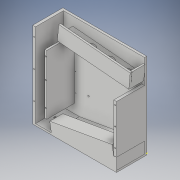
# Autodesk Inventor part: base part
Saved by Autodesk Inventor 2019 (Build 230136000, 136)
## iProperties
Created: 2020-02-20
Part Number: base part
Material: Generic
Document SubType Name: Modeling
Designer: LENOVO
Density: 1 g/cm^3
Appearance: Default
Author: LENOVO
Autodesk Inventor part; units mm, degrees
ref_plane "YZ Plane" through (0, 0, 0) normal (1, 0, 0) x (0, 1, 0)
ref_plane "XZ Plane" through (0, 0, 0) normal (0, 1, 0) x (-1, 0, 0)
ref_plane "XY Plane" through (0, 0, 0) normal (0, 0, 1) x (1, 0, 0)
sketch "Sketch1" plane through (0, 0, 0) normal (0, 0, 1) x (1, 0, 0)
  line L0 (0, 0) -> (450, 0)
  line L1 (450, 0) -> (450, 450)
  line L2 (450, 450) -> (0, 450)
  line L3 (0, 450) -> (0, 0)
  dimension "d0" = 450
  dimension "d1" = 450
  constraints: 8 end point, 2 parallel, 1 horizontal, 1 perpendicular
  measures "d0" distance of L2.end L1.end
  measures "d1" distance of L1.end L0.end
extrude "Extrusion1" add sketch "Sketch1" along normal blind 12
sketch "Sketch2" plane through (0, 0, 12) normal (0, 0, 1) x (1, 0, 0)
  line L0 (100, 400) -> (448.6681, 369.4955)
  line L1 (100, 400) -> (450, 400) construction
  line L2 (448.6681, 369.4955) -> (446.0535, 339.6096)
  line L3 (446.0535, 339.6096) -> (97.3853, 370.1142)
  line L4 (97.3853, 370.1142) -> (100, 400)
  point P0 (0, 0)
  dimension "d4" = 350
  dimension "d5" = 5
  dimension "d6" = 30
  dimension "d7" = 350
  constraints: 10 end point, 2 perpendicular, 1 equal length, 1 horizontal
  measures "d4" distance of L0.start L0.end
  measures "d5" angle of L0 L1
  measures "d6" distance of L0.end L2.end
  measures "d7" distance of L2.end L3.end
extrude "Extrusion2" add sketch "Sketch2" along normal blind 80
sketch "Sketch3" plane through (100, 400, 92) normal (0.0871557, 0.9961947, 0) x (0.9961947, -0.0871557, 0)
  circle A0 centre (100, 40) radius 25
  circle A1 centre (300, 40) radius 25
  circle A2 centre (200, 40) radius 25
  point P0 (-64.7572, 92)
  dimension "d10" = 50
  dimension "d11" = 50
  dimension "d12" = 50
  constraints: 3 centre point
  measures "d10" diameter of A0
  measures "d11" diameter of A1
  measures "d12" diameter of A2
extrude "Extrusion3" cut sketch "Sketch3" against normal blind 80
sketch "Sketch4" plane through (100, 400, 92) normal (0.0871557, 0.9961947, 0) x (0.9961947, -0.0871557, 0)
  line L0 (350, 0) -> (0, 0) projected
  line L1 (0, 0) -> (350, 0)
  line L2 (350, 0) -> (350, 10)
  line L3 (350, 10) -> (0, 10)
  line L4 (0, 10) -> (0, 0)
  point P0 (-64.7572, 92)
  dimension "d15" = 350
  dimension "d16" = 10
  constraints: 8 end point, 2 parallel, 1 horizontal, 1 perpendicular
  measures "d15" distance of L3.end L2.end
  measures "d16" distance of L2.end L1.end
extrude "Extrusion4" add sketch "Sketch4" along normal blind 50
sketch "Sketch5" plane through (0, 0, 0) normal (0, 0, -1) x (-1, 0, 0)
  point P0 (0, 0)
sketch "Sketch6" plane through (0, 0, 12) normal (0, 0, 1) x (1, 0, 0)
  circle A0 centre (135, 350) radius 6.5
  circle A1 centre (240, 345) radius 6.5
  circle A2 centre (340, 340) radius 6.5
  point P0 (0, 0)
  dimension "d19" = 13
  dimension "d20" = 13
  dimension "d21" = 13
  constraints: 3 centre point
  measures "d19" diameter of A0
  measures "d20" diameter of A1
  measures "d21" diameter of A2
extrude "Extrusion5" cut sketch "Sketch6" against normal blind 50
sketch "Sketch7" plane through (448.6681, 369.4955, 82) normal (0.0871557, 0.9961947, 0) x (0.9961947, -0.0871557, 0)
  line L0 (0, 70) -> (0, -10) projected
  line L1 (0, 0.4476) -> (-8.4239, 0.4476)
  line L2 (-8.4239, 0.4476) -> (-8.4239, 70)
  line L3 (-8.4239, 70) -> (0, 70)
  line L4 (0, 70) -> (0, 0.4476)
  point P0 (-414.7572, 82)
  constraints: 8 end point, 2 parallel, 1 horizontal, 1 perpendicular, 1 point on line
extrude "Extrusion6" add sketch "Sketch7" along normal blind 50
sketch "Sketch8" plane through (0, 0, 12) normal (0, 0, 1) x (1, 0, 0)
  line L0 (0, 0) -> (450, 0)
  line L1 (450, 0) -> (450, -50)
  line L2 (450, -50) -> (0, -50)
  line L3 (0, -50) -> (0, 0)
  dimension "d26" = 450
  dimension "d27" = 50
  constraints: 8 end point, 2 parallel, 1 horizontal, 1 perpendicular
  measures "d26" distance of L1.end L2.end
  measures "d27" distance of L0.end L1.end
extrude "Extrusion7" add sketch "Sketch8" against normal blind 12
sketch "Sketch9" plane through (0, 0, 12) normal (0, 0, 1) x (1, 0, 0)
  line L0 (450, 450) -> (0, 450) projected
  line L1 (100, 450) -> (100, 0)
  line L2 (100, 0) -> (449.6068, 61.6451)
  line L3 (449.6068, 61.6451) -> (449.6068, 0)
  line L4 (449.6068, 0) -> (100, 0)
  point P0 (0, 0)
  dimension "d30" = 355
  dimension "d31" = 80
  dimension "d32" = 80
  constraints: 8 end point, 1 perpendicular, 1 point on line, 1 vertical
  measures "d30" distance of L1.end L2.end
  measures "d31" angle of L2 L1
  measures "d32" angle of L2 L3
extrude "Extrusion8" add sketch "Sketch9" along normal blind 85
sketch "Sketch10" plane through (0, 0, 12) normal (0, 0, 1) x (1, 0, 0)
  line L0 (450, -50) -> (0, -50) projected
  line L1 (0, 0) -> (450, 0)
  line L2 (450, 0) -> (450, -50)
  line L3 (450, -50) -> (0, -50)
  line L4 (0, -50) -> (0, 0)
  constraints: 8 end point, 2 parallel, 1 horizontal, 1 perpendicular
sketch "Sketch11" plane through (0, 0, 97) normal (0, 0, 1) x (1, 0, 0)
  line L0 (100, 0) -> (449.6068, 0) projected
  line L1 (449.6068, 61.6451) -> (100, 0) projected
  line L2 (100, 0) -> (449.6068, 61.6451)
  line L3 (449.6068, 61.6451) -> (449.6068, 0)
  line L4 (449.6068, 0) -> (100, 0)
  point P0 (0, 0)
  constraints: 6 end point, 1 collinear, 1 perpendicular, 1 vertical
extrude "Extrusion9" add sketch "Sketch11" along normal blind 65
extrude "Extrusion10" add sketch "Sketch10" along normal blind 150
sketch "Sketch12" plane through (0, 0, 12) normal (0, 0, 1) x (1, 0, 0)
  line L0 (0, 450) -> (0, -50) projected
  line L1 (0, 0) -> (100, 0) projected
  line L2 (0, 450) -> (15, 450)
  line L3 (15, 450) -> (15, 0)
  line L4 (15, 0) -> (0, 0)
  line L5 (0, 0) -> (0, 450)
  line L6 (450, 384.7187) -> (450, 0) projected
  line L7 (450, 320) -> (435, 320)
  line L8 (435, 320) -> (435, 61)
  line L9 (435, 61) -> (450, 61)
  line L10 (450, 61) -> (450, 320)
  dimension "d39" = 15
  dimension "d40" = 15
  dimension "d41" = 259
  constraints: 16 end point, 4 parallel, 2 horizontal, 2 perpendicular, 2 point on line
  measures "d39" distance of L3.end L4.end
  measures "d40" distance of L9.end L8.end
  measures "d41" distance of L8.end L7.end
extrude "Extrusion11" add sketch "Sketch12" along normal blind 150
sketch "Sketch13" plane through (449.6068, 0, 162) normal (1, 0, 0) x (0, 0, -1)
  line L0 (150, 0) -> (0, 0) projected
  line L1 (150, 61) -> (0, 61) projected
  line L2 (0, 0) -> (150, 0)
  line L3 (150, 0) -> (150, 61)
  line L4 (150, 61) -> (0, 61)
  line L5 (0, 61) -> (0, 0)
  point P0 (162, 0)
  constraints: 8 end point, 2 parallel, 1 horizontal, 1 perpendicular
extrude "Extrusion12" add sketch "Sketch13" along normal blind 0.4
sketch "Sketch14" plane through (0, 0, 12) normal (0, 0, 1) x (1, 0, 0)
  line L0 (75, 370) -> (65, 370)
  line L1 (65, 370) -> (65, 50)
  line L2 (65, 50) -> (75, 50)
  line L3 (75, 50) -> (75, 370)
  point P0 (0, 0)
  dimension "d46" = 10
  dimension "d47" = 320
  constraints: 8 end point, 2 parallel, 1 horizontal, 1 perpendicular
  measures "d46" distance of L2.end L1.end
  measures "d47" distance of L1.end L0.end
extrude "Extrusion13" add sketch "Sketch14" along normal blind 150
sketch "Sketch15" plane through (100, 0, 162) normal (0, 1, 0) x (1, 0, 0)
  circle A0 centre (-60, 81) radius 6.5
  point P0 (-100, 162)
  dimension "d50" = 13
  constraints: 1 centre point
  measures "d50" diameter of A0
extrude "Extrusion14" cut sketch "Sketch15" against normal blind 150
thread "Thread1" size "M14x2" class "6H" standard "ANSI Metric M Profile" full length
sketch "Sketch16" plane through (100, 0, 162) normal (-0.1736482, 0.9848078, 0) x (0.9848078, 0.1736482, 0)
  line L0 (0, 150) -> (0, 0) projected
  line L1 (0, 0) -> (340, 0)
  line L2 (340, 0) -> (340, 70)
  line L3 (340, 70) -> (0, 70)
  line L4 (0, 70) -> (0, 0)
  point P0 (-98.4808, 162)
  dimension "d55" = 340
  dimension "d56" = 70
  constraints: 8 end point, 2 parallel, 1 horizontal, 1 perpendicular
  measures "d55" distance of L3.end L2.end
  measures "d56" distance of L2.end L1.end
extrude "Extrusion15" add sketch "Sketch16" along normal blind 50
sketch "Sketch17" plane through (0, -50, 0) normal (0, -1, 0) x (1, 0, 0)
  line L0 (450, 0) -> (0, 0) projected
  line L1 (0, 0) -> (450, 0)
  line L2 (450, 0) -> (450, 162)
  line L3 (450, 162) -> (0, 162)
  line L4 (0, 162) -> (0, 0)
  dimension "d59" = 450
  constraints: 8 end point, 2 parallel, 1 horizontal, 1 perpendicular
  measures "d59" distance of L3.end L2.end
extrude "Extrusion16" cut sketch "Sketch17" against normal blind 20
sketch "Sketch18" plane through (0, -30, 0) normal (0, -1, 0) x (1, 0, 0)
  line L0 (0, 0) -> (450, 0)
  line L1 (450, 0) -> (450, 162)
  line L2 (450, 162) -> (0, 162)
  line L3 (0, 162) -> (0, 0)
  dimension "d62" = 450
  dimension "d63" = 162
  constraints: 8 end point, 2 parallel, 1 horizontal, 1 perpendicular
  measures "d62" distance of L2.end L1.end
  measures "d63" distance of L1.end L0.end
extrude "Extrusion17" cut sketch "Sketch18" against normal blind 10
sketch "Sketch19" plane through (0, -20, 0) normal (0, -1, 0) x (1, 0, 0)
  line L0 (450, 12) -> (450, 162) projected
  line L1 (0, 0) -> (450, 0)
  line L2 (450, 0) -> (450, 162)
  line L3 (450, 162) -> (0, 162)
  line L4 (0, 162) -> (0, 0)
  constraints: 8 end point, 2 parallel, 1 horizontal, 1 perpendicular
extrude "Extrusion18" cut sketch "Sketch19" against normal blind 10
sketch "Sketch20" plane through (0, 0, 162) normal (0, 0, 1) x (1, 0, 0)
  circle A0 centre (70, 340) radius 3
  circle A1 centre (70, 100) radius 3
  circle A2 centre (70, 230) radius 3
  point P0 (0, 0)
  dimension "d68" = 6
  dimension "d69" = 6
  dimension "d70" = 6
  constraints: 3 centre point
  measures "d68" diameter of A0
  measures "d69" diameter of A1
  measures "d70" diameter of A2
extrude "Extrusion19" cut sketch "Sketch20" against normal blind 10
thread "Thread2" size "M6x1" class "6H" standard "ANSI Metric M Profile" full length
thread "Thread3" size "M6x1" class "6H" standard "ANSI Metric M Profile" full length
thread "Thread4" size "M6x1" class "6H" standard "ANSI Metric M Profile" full length
sketch "Sketch21" plane through (0, 0, 0) normal (0, 0, -1) x (-1, 0, 0)
  circle A0 centre (-70, 340) radius 3 projected
  circle A1 centre (-70, 340) radius 3
  circle A2 centre (-70, 230) radius 3 projected
  circle A3 centre (-70, 230) radius 3
  circle A4 centre (-70, 100) radius 3 projected
  circle A5 centre (-70, 100) radius 3
  point P0 (0, 0)
  dimension "d79" = 6
  dimension "d80" = 6
  dimension "d81" = 6
  constraints: 3 centre point, 3 coincident
  measures "d79" diameter of A1
  measures "d80" diameter of A3
  measures "d81" diameter of A5
extrude "Extrusion20" cut sketch "Sketch21" against normal blind 20
thread "Thread5" size "M6x1" class "6H" standard "ANSI Metric M Profile" full length
thread "Thread6" size "M6x1" class "6H" standard "ANSI Metric M Profile" full length
thread "Thread7" size "M6x1" class "6H" standard "ANSI Metric M Profile" full length
sketch "Sketch22" plane through (0, 0, 0) normal (0, 0, -1) x (-1, 0, 0)
  circle A0 centre (-7.5, 100) radius 3
  circle A1 centre (-7.5, 250) radius 3
  circle A2 centre (-7.5, 400) radius 3
  point P0 (0, 0)
  dimension "d90" = 6
  dimension "d91" = 6
  dimension "d92" = 6
  constraints: 3 centre point
  measures "d90" diameter of A0
  measures "d91" diameter of A1
  measures "d92" diameter of A2
extrude "Extrusion21" cut sketch "Sketch22" against normal blind 20
thread "Thread8" size "M6x1" class "6H" standard "ANSI Metric M Profile" full length
thread "Thread9" size "M6x1" class "6H" standard "ANSI Metric M Profile" full length
thread "Thread10" size "M6x1" class "6H" standard "ANSI Metric M Profile" full length
sketch "Sketch23" plane through (0, 0, 162) normal (0, 0, 1) x (1, 0, 0)
  circle A0 centre (7.5, 100) radius 3
  circle A1 centre (7.5, 250) radius 3
  circle A2 centre (7.5, 400) radius 3
  point P0 (0, 0)
  dimension "d101" = 6
  dimension "d102" = 6
  dimension "d103" = 6
  constraints: 3 centre point
  measures "d101" diameter of A0
  measures "d102" diameter of A1
  measures "d103" diameter of A2
extrude "Extrusion22" cut sketch "Sketch23" against normal blind 20
sketch "Sketch24" plane through (0, 0, 162) normal (0, 0, 1) x (1, 0, 0)
  circle A0 centre (442.5, 100) radius 3
  circle A1 centre (442.5, 300) radius 3
  circle A2 centre (442.5, 200) radius 3
  point P0 (0, 0)
  dimension "d106" = 6
  dimension "d107" = 6
  dimension "d108" = 6
  constraints: 3 centre point
  measures "d106" diameter of A0
  measures "d107" diameter of A1
  measures "d108" diameter of A2
extrude "Extrusion23" cut sketch "Sketch24" against normal blind 20
thread "Thread11" size "M6x1" class "6H" standard "ANSI Metric M Profile" full length
thread "Thread12" size "M6x1" class "6H" standard "ANSI Metric M Profile" full length
thread "Thread13" size "M6x1" class "6H" standard "ANSI Metric M Profile" full length
thread "Thread14" size "M6x1" class "6H" standard "ANSI Metric M Profile" full length
sketch "Sketch25" plane through (0, 0, 0) normal (0, 0, -1) x (-1, 0, 0)
  circle A0 centre (-442.5, 100) radius 3
  circle A1 centre (-442.5, 200) radius 3
  circle A2 centre (-442.5, 300) radius 3
  point P0 (0, 0)
  dimension "d119" = 6
  dimension "d120" = 6
  dimension "d121" = 6
  constraints: 3 centre point
  measures "d119" diameter of A0
  measures "d120" diameter of A1
  measures "d121" diameter of A2
extrude "Extrusion24" cut sketch "Sketch25" against normal blind 20
thread "Thread15" size "M6x1" class "6H" standard "ANSI Metric M Profile" full length
thread "Thread16" size "M6x1" class "6H" standard "ANSI Metric M Profile" full length
thread "Thread17" size "M6x1" class "6H" standard "ANSI Metric M Profile" full length
sketch "Sketch26" plane through (0, 0, 0) normal (0, 0, -1) x (-1, 0, 0)
  point P0 (0, 0)
sketch "Sketch27" plane through (0, -10, 0) normal (0, -1, 0) x (1, 0, 0)
  circle A0 centre (114.2728, 152.7647) radius 3
  circle A1 centre (256.2116, 149.7647) radius 3
  circle A2 centre (406.5706, 149.7647) radius 3
  point P0 (0, 0)
  dimension "d130" = 6
  dimension "d131" = 6
  dimension "d132" = 6
  constraints: 3 centre point
  measures "d130" diameter of A0
  measures "d131" diameter of A1
  measures "d132" diameter of A2
extrude "Extrusion25" cut sketch "Sketch27" against normal blind 20
thread "Thread18" size "M6x1" class "6H" standard "ANSI Metric M Profile" full length
thread "Thread19" size "M6x1" class "6H" standard "ANSI Metric M Profile" full length
thread "Thread20" size "M6x1" class "6H" standard "ANSI Metric M Profile" full length
sketch "Sketch28" plane through (446.0535, 339.6096, 12) normal (-0.0871557, -0.9961947, 0) x (0.9961947, -0.0871557, 0)
  circle A0 centre (-336.1769, 75.2704) radius 3
  circle A1 centre (-277.2392, 75.2704) radius 3
  circle A2 centre (-192.8045, 66.3693) radius 3
  circle A3 centre (-86.956, 63.3693) radius 3
  point P0 (-414.7572, -12)
  dimension "d141" = 6
  dimension "d142" = 6
  dimension "d143" = 6
  dimension "d144" = 6
  constraints: 4 centre point
  measures "d141" diameter of A0
  measures "d142" diameter of A1
  measures "d143" diameter of A2
  measures "d144" diameter of A3
extrude "Extrusion26" cut sketch "Sketch28" against normal blind 20
thread "Thread21" size "M6x1" class "6H" standard "ANSI Metric M Profile" full length
thread "Thread22" size "M6x1" class "6H" standard "ANSI Metric M Profile" full length
thread "Thread23" size "M6x1" class "6H" standard "ANSI Metric M Profile" full length
thread "Thread24" size "M6x1" class "6H" standard "ANSI Metric M Profile" full length
thread "Thread25" size "M6x1" class "6H" standard "ANSI Metric M Profile" full length
thread "Thread26" size "M6x1" class "6H" standard "ANSI Metric M Profile" full length
sketch "Sketch29" plane through (0, 0, 0) normal (0, 0, -1) x (-1, 0, 0)
  point P0 (0, 0)
sketch "Sketch30" plane through (0, 0, 12) normal (0, 0, 1) x (1, 0, 0)
  point P0 (0, 0)
sketch "Sketch31" plane through (450, 384.7187, 12) normal (1, 0, 0) x (0, 0, -1)
  point P0 (12, -384.7187)
sketch "Sketch32" plane through (0, 0, 0) normal (0, 0, -1) x (-1, 0, 0)
  circle A0 centre (-340, 230) radius 4
  point P0 (0, 0)
  dimension "d159" = 8
  constraints: 1 centre point
  measures "d159" diameter of A0
extrude "Extrusion27" cut sketch "Sketch32" against normal blind 30
sketch "Sketch33" plane through (0, 0, 0) normal (0, 0, -1) x (-1, 0, 0)
  circle A0 centre (-380, 230) radius 4
  point P0 (0, 0)
  dimension "d162" = 8
  constraints: 1 centre point
  measures "d162" diameter of A0
extrude "Extrusion28" cut sketch "Sketch33" against normal blind 30
sketch "Sketch34" plane through (0, 0, 0) normal (0, 0, -1) x (-1, 0, 0)
  circle A0 centre (-400, 200) radius 4
  point P0 (0, 0)
  dimension "d165" = 8
  constraints: 1 centre point
  measures "d165" diameter of A0
extrude "Extrusion29" cut sketch "Sketch34" against normal blind 30
sketch "Sketch35" plane through (0, 0, 12) normal (0, 0, 1) x (1, 0, 0)
  circle A0 centre (81, 100) radius 1.5
  point P0 (0, 0)
  dimension "d168" = 3
  constraints: 1 centre point
  measures "d168" diameter of A0
extrude "Extrusion30" cut sketch "Sketch35" against normal blind 30
sketch "Sketch36" plane through (0, 0, 12) normal (0, 0, 1) x (1, 0, 0)
  circle A0 centre (81, 200) radius 1.5
  circle A1 centre (81, 300) radius 4
  point P0 (0, 0)
  dimension "d171" = 3
  dimension "d172" = 8
  constraints: 2 centre point
  measures "d171" diameter of A0
  measures "d172" diameter of A1
extrude "Extrusion31" cut sketch "Sketch36" against normal blind 30
sketch "Sketch37" plane through (0, 0, 0) normal (0, 0, -1) x (-1, 0, 0)
  point P0 (0, 0)
sketch "Sketch38" plane through (0, 0, 0) normal (0, 0, -1) x (-1, 0, 0)
  point P0 (0, 0)
sketch "Sketch39" plane through (0, 0, 12) normal (0, 0, 1) x (1, 0, 0)
  point P0 (0, 0)
sketch "Sketch40" plane through (0, 0, 12) normal (0, 0, 1) x (1, 0, 0)
  circle A0 centre (429, 300) radius 1.5
  circle A1 centre (3, 200) radius 1.5
  circle A2 centre (429, 200) radius 1.5
  circle A3 centre (429, 140) radius 1.5
  point P0 (0, 0)
  dimension "d175" = 3
  dimension "d176" = 3
  dimension "d177" = 3
  dimension "d178" = 3
  constraints: 4 centre point
  measures "d175" diameter of A0
  measures "d176" diameter of A1
  measures "d177" diameter of A2
  measures "d178" diameter of A3
extrude "Extrusion32" cut sketch "Sketch40" against normal blind 20 contours A0 | A2 | A3
sketch "Sketch41" plane through (0, 0, 12) normal (0, 0, 1) x (1, 0, 0)
  point P0 (0, 0)
sketch "Sketch42" plane through (15, 0, 12) normal (1, 0, 0) x (0, 0, -1)
  point P0 (12, 0)
sketch "Sketch43" plane through (0, 0, 12) normal (0, 0, 1) x (1, 0, 0)
  circle A0 centre (21, 100) radius 1.5
  circle A1 centre (21, 200) radius 1.5
  circle A2 centre (21, 350) radius 1.5
  point P0 (0, 0)
  dimension "d181" = 3
  dimension "d182" = 3
  dimension "d183" = 3
  constraints: 3 centre point
  measures "d181" diameter of A0
  measures "d182" diameter of A1
  measures "d183" diameter of A2
extrude "Extrusion33" cut sketch "Sketch43" against normal blind 20
sketch "Sketch44" plane through (0, 0, 0) normal (0, 0, -1) x (-1, 0, 0)
  circle A0 centre (-150, 200) radius 4
  point P0 (0, 0)
  dimension "d186" = 8
  constraints: 1 centre point
  measures "d186" diameter of A0
extrude "Extrusion34" cut sketch "Sketch44" against normal blind 30
sketch "Sketch45" plane through (0, 0, 0) normal (0, 0, -1) x (-1, 0, 0)
  circle A0 centre (-150, 120) radius 4
  point P0 (0, 0)
  dimension "d189" = 8
  constraints: 1 centre point
  measures "d189" diameter of A0
extrude "Extrusion35" cut sketch "Sketch45" against normal blind 30
sketch "Sketch46" plane through (0, 0, 0) normal (0, 0, -1) x (-1, 0, 0)
  circle A0 centre (-150, 200) radius 4 projected
  circle A1 centre (-150, 200) radius 4
  point P0 (0, 0)
  dimension "d192" = 8
  constraints: 1 centre point, 1 coincident
  measures "d192" diameter of A1
extrude "Extrusion36" add sketch "Sketch46" against normal blind 12
sketch "Sketch47" plane through (0, 0, 0) normal (0, 0, -1) x (-1, 0, 0)
  circle A0 centre (-380, 230) radius 4 projected
  circle A1 centre (-380, 230) radius 4
  circle A2 centre (-340, 230) radius 4 projected
  circle A3 centre (-340, 230) radius 4
  point P0 (0, 0)
  dimension "d195" = 8
  dimension "d196" = 8
  constraints: 2 centre point, 2 coincident
  measures "d195" diameter of A1
  measures "d196" diameter of A3
extrude "Extrusion37" add sketch "Sketch47" against normal blind 12
sketch "Sketch48" plane through (97.3853, 370.1142, 12) normal (-0.9961947, 0.0871557, 0) x (0, 0, 1)
  line L0 (0, 0) -> (0, 30) projected
  line L1 (0, 30) -> (70, 30) projected
  line L2 (0, 0) -> (70, 0)
  line L3 (70, 0) -> (70, 30)
  line L4 (70, 30) -> (0, 30)
  line L5 (0, 30) -> (0, 0)
  line L6 (80, 0) -> (80, 80) projected
  line L7 (70, 0) -> (80, 0)
  line L8 (80, 0) -> (80, 80)
  line L9 (80, 80) -> (70, 80)
  line L10 (70, 80) -> (70, 0)
  point P0 (-12, -377.1935)
  constraints: 16 end point, 4 parallel, 2 horizontal, 2 perpendicular
extrude "Extrusion38" add sketch "Sketch48" along normal blind 35
body "Solid1"
